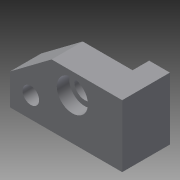
# Autodesk Inventor part: 零件7-21-1
Saved by Autodesk Inventor 2014 (Build 180170000, 170)
## iProperties
Created: 2018-12-21
Part Number: 零件7-21-1
Material: 常规
Document SubType Name: Modeling
Designer: Administrator
Density: 1 g/cm^3
Appearance: 默认
Author: Administrator
Autodesk Inventor part; units mm, degrees
ref_plane "YZ Plane" through (0, 0, 0) normal (1, 0, 0) x (0, 1, 0)
ref_plane "XZ Plane" through (0, 0, 0) normal (0, 1, 0) x (-1, 0, 0)
ref_plane "XY Plane" through (0, 0, 0) normal (0, 0, 1) x (1, 0, 0)
sketch "草图1" plane through (0, 0, 0) normal (0, 1, 0) x (-1, 0, 0)
  line L0 (-27, 15) -> (7, 15)
  line L1 (27, 0) -> (27, -15)
  line L2 (27, -15) -> (-27, -15)
  line L3 (-27, -15) -> (-27, 15)
  line L4 (-27, 15) -> (27, -15) construction
  line L5 (27, 15) -> (-27, -15) construction
  line L6 (27, 0) -> (7, 15)
  circle A0 centre (17, -5) radius 4
  circle A1 centre (-3, 5) radius 5
  point P0 (0, 0)
  dimension "d0" = 54
  dimension "d1" = 30
  dimension "d2" = 20
  dimension "d3" = 8
  dimension "d4" = 10
  dimension "d5" = 10
  dimension "d6" = 10
  dimension "d7" = 20
  dimension "d8" = 30
  constraints: 14 end point, 2 centre point, 2 midpoint, 2 parallel, 1 horizontal, 1 perpendicular
  measures "d0" distance of L1.end L2.end
  measures "d1" distance of L2.end L0.start
  measures "d2" distance of L0.end L5.start
  measures "d3" diameter of A0
  measures "d4" distance from line of L2 A0.centre
  measures "d5" distance from line of L1 A0.centre
  measures "d6" diameter of A1
  measures "d7" distance from line of L2 A1.centre
  measures "d8" distance from line of L1 A1.centre
extrude "拉伸1" add sketch "草图1" along normal blind 15
sketch "草图2" plane through (0, 0, 0) normal (0, 1, 0) x (-1, 0, 0)
  circle A0 centre (-3, 5) radius 5 projected
  circle A1 centre (17, -5) radius 4 projected
  line L0 (7, 15) -> (-27, 15) projected
  line L1 (-27, 15) -> (-27, -15) projected
  line L2 (-27, -15) -> (27, -15) projected
  line L3 (27, -15) -> (27, 0) projected
  line L4 (27, 0) -> (7, 15) projected
  circle A2 centre (-3, 5) radius 7.5
  point P0 (0, 0)
  dimension "d11" = 15
  constraints: 1 centre point, 1 coincident
  measures "d11" diameter of A2
extrude "拉伸2" cut sketch "草图2" along normal blind 6 contours A2
sketch "草图3" plane through (0, 15, 0) normal (0, 1, 0) x (1, 0, 0)
  line L0 (-7, -15) -> (27, -15) projected
  line L1 (27, -15) -> (27, 15) projected
  line L2 (27, 15) -> (-27, 15) projected
  line L3 (17, 15) -> (17, -15)
  point P0 (0, 0)
  dimension "d14" = 10
  constraints: 2 end point, 2 point on line, 1 perpendicular
  measures "d14" distance between parallel lines of L1 L3
extrude "拉伸3" add sketch "草图3" along normal blind 8
hole "孔1" at (22, 23, 10) direction (0, -1, 0) diameter 4 depth 12 tip angle 118
hole "孔2" at (22, 23, -10) direction (0, -1, 0) diameter 4 depth 12 tip angle 118
